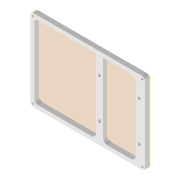
# Autodesk Inventor part: Omniscope_USBC_Base_Bottom
Saved by Autodesk Inventor 2022 (Build 260153000, 153)
## iProperties
Created: 2023-05-17
Part Number: Omniscope_USBC_Base_Bottom
Material: Generisch
Document SubType Name: Modeling
Designer: diederichbenedict
Density: 1 g/cm^3
Appearance: Vorgabe
Author: diederichbenedict
Autodesk Inventor part; units mm, degrees
(part 1 of 3)
ref_plane "YZ Plane" through (0, 0, 0) normal (1, 0, 0) x (0, 1, 0)
ref_plane "XZ Plane" through (0, 0, 0) normal (0, 1, 0) x (-1, 0, 0)
ref_plane "XY Plane" through (0, 0, 0) normal (0, 0, 1) x (1, 0, 0)
ref_plane "Arbeitsebene1" through (0, 0, 0) normal (0, 0, 1) x (1, 0, 0)
sketch "Skizze1" plane through (0, 0, 0) normal (0, 0, 1) x (1, 0, 0)
  line L0 (-66.421, 45.4152) -> (66.421, 45.4152)
  line L1 (-66.421, -45.4152) -> (-66.421, 45.4152)
  line L2 (66.421, -45.4152) -> (-66.421, -45.4152)
  line L3 (66.421, 45.4152) -> (66.421, -45.4152)
  line L4 (44.2834, -26.0546) -> (45.8834, -26.0546)
  line L5 (44.2834, -25.4046) -> (44.2834, -26.0546)
  line L6 (45.8834, -25.4046) -> (44.2834, -25.4046)
  line L7 (45.8834, -26.0546) -> (45.8834, -25.4046)
  line L8 (44.2834, -33.9546) -> (45.8834, -33.9546)
  line L9 (44.2834, -33.3046) -> (44.2834, -33.9546)
  line L10 (45.8834, -33.3046) -> (44.2834, -33.3046)
  line L11 (45.8834, -33.9546) -> (45.8834, -33.3046)
  line L12 (43.4184, -27.0796) -> (44.2084, -27.0796)
  line L13 (43.4184, -26.6796) -> (43.4184, -27.0796)
  line L14 (44.2084, -26.6796) -> (43.4184, -26.6796)
  line L15 (44.2084, -27.0796) -> (44.2084, -26.6796)
  line L16 (45.9584, -27.0796) -> (46.7484, -27.0796)
  line L17 (45.9584, -26.6796) -> (45.9584, -27.0796)
  line L18 (46.7484, -26.6796) -> (45.9584, -26.6796)
  line L19 (46.7484, -27.0796) -> (46.7484, -26.6796)
  line L20 (43.4184, -27.8796) -> (44.2084, -27.8796)
  line L21 (43.4184, -27.4796) -> (43.4184, -27.8796)
  line L22 (44.2084, -27.4796) -> (43.4184, -27.4796)
  line L23 (44.2084, -27.8796) -> (44.2084, -27.4796)
  line L24 (45.9584, -27.8796) -> (46.7484, -27.8796)
  line L25 (45.9584, -27.4796) -> (45.9584, -27.8796)
  line L26 (46.7484, -27.4796) -> (45.9584, -27.4796)
  line L27 (46.7484, -27.8796) -> (46.7484, -27.4796)
  line L28 (43.4184, -28.6796) -> (44.2084, -28.6796)
  line L29 (43.4184, -28.2796) -> (43.4184, -28.6796)
  line L30 (44.2084, -28.2796) -> (43.4184, -28.2796)
  line L31 (44.2084, -28.6796) -> (44.2084, -28.2796)
  line L32 (45.9584, -28.6796) -> (46.7484, -28.6796)
  line L33 (45.9584, -28.2796) -> (45.9584, -28.6796)
  line L34 (46.7484, -28.2796) -> (45.9584, -28.2796)
  line L35 (46.7484, -28.6796) -> (46.7484, -28.2796)
  line L36 (43.4184, -29.4796) -> (44.2084, -29.4796)
  line L37 (43.4184, -29.0796) -> (43.4184, -29.4796)
  line L38 (44.2084, -29.0796) -> (43.4184, -29.0796)
  line L39 (44.2084, -29.4796) -> (44.2084, -29.0796)
  line L40 (45.9584, -29.4796) -> (46.7484, -29.4796)
  line L41 (45.9584, -29.0796) -> (45.9584, -29.4796)
  line L42 (46.7484, -29.0796) -> (45.9584, -29.0796)
  line L43 (46.7484, -29.4796) -> (46.7484, -29.0796)
  line L44 (43.4184, -30.2796) -> (44.2084, -30.2796)
  line L45 (43.4184, -29.8796) -> (43.4184, -30.2796)
  line L46 (44.2084, -29.8796) -> (43.4184, -29.8796)
  line L47 (44.2084, -30.2796) -> (44.2084, -29.8796)
  line L48 (45.9584, -30.2796) -> (46.7484, -30.2796)
  line L49 (45.9584, -29.8796) -> (45.9584, -30.2796)
  line L50 (46.7484, -29.8796) -> (45.9584, -29.8796)
  line L51 (46.7484, -30.2796) -> (46.7484, -29.8796)
  line L52 (43.4184, -31.0796) -> (44.2084, -31.0796)
  line L53 (43.4184, -30.6796) -> (43.4184, -31.0796)
  line L54 (44.2084, -30.6796) -> (43.4184, -30.6796)
  line L55 (44.2084, -31.0796) -> (44.2084, -30.6796)
  line L56 (45.9584, -31.0796) -> (46.7484, -31.0796)
  line L57 (45.9584, -30.6796) -> (45.9584, -31.0796)
  line L58 (46.7484, -30.6796) -> (45.9584, -30.6796)
  line L59 (46.7484, -31.0796) -> (46.7484, -30.6796)
  line L60 (43.4184, -31.8796) -> (44.2084, -31.8796)
  line L61 (43.4184, -31.4796) -> (43.4184, -31.8796)
  line L62 (44.2084, -31.4796) -> (43.4184, -31.4796)
  line L63 (44.2084, -31.8796) -> (44.2084, -31.4796)
  line L64 (45.9584, -31.8796) -> (46.7484, -31.8796)
  line L65 (45.9584, -31.4796) -> (45.9584, -31.8796)
  line L66 (46.7484, -31.4796) -> (45.9584, -31.4796)
  line L67 (46.7484, -31.8796) -> (46.7484, -31.4796)
  line L68 (43.4184, -32.6796) -> (44.2084, -32.6796)
  line L69 (43.4184, -32.2796) -> (43.4184, -32.6796)
  line L70 (44.2084, -32.2796) -> (43.4184, -32.2796)
  line L71 (44.2084, -32.6796) -> (44.2084, -32.2796)
  line L72 (45.9584, -32.6796) -> (46.7484, -32.6796)
  line L73 (45.9584, -32.2796) -> (45.9584, -32.6796)
  line L74 (46.7484, -32.2796) -> (45.9584, -32.2796)
  line L75 (46.7484, -32.6796) -> (46.7484, -32.2796)
  line L76 (-29.4941, -14.7296) -> (-31.0941, -14.7296)
  line L77 (-29.4941, -15.3796) -> (-29.4941, -14.7296)
  line L78 (-31.0941, -15.3796) -> (-29.4941, -15.3796)
  line L79 (-31.0941, -14.7296) -> (-31.0941, -15.3796)
  line L80 (-29.4941, -6.8296) -> (-31.0941, -6.8296)
  line L81 (-29.4941, -7.4796) -> (-29.4941, -6.8296)
  line L82 (-31.0941, -7.4796) -> (-29.4941, -7.4796)
  line L83 (-31.0941, -6.8296) -> (-31.0941, -7.4796)
  line L84 (-28.6291, -13.7046) -> (-29.4191, -13.7046)
  line L85 (-28.6291, -14.1046) -> (-28.6291, -13.7046)
  line L86 (-29.4191, -14.1046) -> (-28.6291, -14.1046)
  line L87 (-29.4191, -13.7046) -> (-29.4191, -14.1046)
  line L88 (-31.1691, -13.7046) -> (-31.9591, -13.7046)
  line L89 (-31.1691, -14.1046) -> (-31.1691, -13.7046)
  line L90 (-31.9591, -14.1046) -> (-31.1691, -14.1046)
  line L91 (-31.9591, -13.7046) -> (-31.9591, -14.1046)
  line L92 (-28.6291, -12.9046) -> (-29.4191, -12.9046)
  line L93 (-28.6291, -13.3046) -> (-28.6291, -12.9046)
  line L94 (-29.4191, -13.3046) -> (-28.6291, -13.3046)
  line L95 (-29.4191, -12.9046) -> (-29.4191, -13.3046)
  line L96 (-31.1691, -12.9046) -> (-31.9591, -12.9046)
  line L97 (-31.1691, -13.3046) -> (-31.1691, -12.9046)
  line L98 (-31.9591, -13.3046) -> (-31.1691, -13.3046)
  line L99 (-31.9591, -12.9046) -> (-31.9591, -13.3046)
  line L100 (-28.6291, -12.1046) -> (-29.4191, -12.1046)
  line L101 (-28.6291, -12.5046) -> (-28.6291, -12.1046)
  line L102 (-29.4191, -12.5046) -> (-28.6291, -12.5046)
  line L103 (-29.4191, -12.1046) -> (-29.4191, -12.5046)
  line L104 (-31.1691, -12.1046) -> (-31.9591, -12.1046)
  line L105 (-31.1691, -12.5046) -> (-31.1691, -12.1046)
  line L106 (-31.9591, -12.5046) -> (-31.1691, -12.5046)
  line L107 (-31.9591, -12.1046) -> (-31.9591, -12.5046)
  line L108 (-28.6291, -11.3046) -> (-29.4191, -11.3046)
  line L109 (-28.6291, -11.7046) -> (-28.6291, -11.3046)
  line L110 (-29.4191, -11.7046) -> (-28.6291, -11.7046)
  line L111 (-29.4191, -11.3046) -> (-29.4191, -11.7046)
  line L112 (-31.1691, -11.3046) -> (-31.9591, -11.3046)
  line L113 (-31.1691, -11.7046) -> (-31.1691, -11.3046)
  line L114 (-31.9591, -11.7046) -> (-31.1691, -11.7046)
  line L115 (-31.9591, -11.3046) -> (-31.9591, -11.7046)
  line L116 (-28.6291, -10.5046) -> (-29.4191, -10.5046)
  line L117 (-28.6291, -10.9046) -> (-28.6291, -10.5046)
  line L118 (-29.4191, -10.9046) -> (-28.6291, -10.9046)
  line L119 (-29.4191, -10.5046) -> (-29.4191, -10.9046)
  line L120 (-31.1691, -10.5046) -> (-31.9591, -10.5046)
  line L121 (-31.1691, -10.9046) -> (-31.1691, -10.5046)
  line L122 (-31.9591, -10.9046) -> (-31.1691, -10.9046)
  line L123 (-31.9591, -10.5046) -> (-31.9591, -10.9046)
  line L124 (-28.6291, -9.7046) -> (-29.4191, -9.7046)
  line L125 (-28.6291, -10.1046) -> (-28.6291, -9.7046)
  line L126 (-29.4191, -10.1046) -> (-28.6291, -10.1046)
  line L127 (-29.4191, -9.7046) -> (-29.4191, -10.1046)
  line L128 (-31.1691, -9.7046) -> (-31.9591, -9.7046)
  line L129 (-31.1691, -10.1046) -> (-31.1691, -9.7046)
  line L130 (-31.9591, -10.1046) -> (-31.1691, -10.1046)
  line L131 (-31.9591, -9.7046) -> (-31.9591, -10.1046)
  line L132 (-28.6291, -8.9046) -> (-29.4191, -8.9046)
  line L133 (-28.6291, -9.3046) -> (-28.6291, -8.9046)
  line L134 (-29.4191, -9.3046) -> (-28.6291, -9.3046)
  line L135 (-29.4191, -8.9046) -> (-29.4191, -9.3046)
  line L136 (-31.1691, -8.9046) -> (-31.9591, -8.9046)
  line L137 (-31.1691, -9.3046) -> (-31.1691, -8.9046)
  line L138 (-31.9591, -9.3046) -> (-31.1691, -9.3046)
  line L139 (-31.9591, -8.9046) -> (-31.9591, -9.3046)
  line L140 (-28.6291, -8.1046) -> (-29.4191, -8.1046)
  line L141 (-28.6291, -8.5046) -> (-28.6291, -8.1046)
  line L142 (-29.4191, -8.5046) -> (-28.6291, -8.5046)
  line L143 (-29.4191, -8.1046) -> (-29.4191, -8.5046)
  line L144 (-31.1691, -8.1046) -> (-31.9591, -8.1046)
  line L145 (-31.1691, -8.5046) -> (-31.1691, -8.1046)
  line L146 (-31.9591, -8.5046) -> (-31.1691, -8.5046)
  line L147 (-31.9591, -8.1046) -> (-31.9591, -8.5046)
  line L148 (-10.6116, 22.9704) -> (-12.2116, 22.9704)
  line L149 (-10.6116, 22.3204) -> (-10.6116, 22.9704)
  line L150 (-12.2116, 22.3204) -> (-10.6116, 22.3204)
  line L151 (-12.2116, 22.9704) -> (-12.2116, 22.3204)
  line L152 (-10.6116, 30.8704) -> (-12.2116, 30.8704)
  line L153 (-10.6116, 30.2204) -> (-10.6116, 30.8704)
  line L154 (-12.2116, 30.2204) -> (-10.6116, 30.2204)
  line L155 (-12.2116, 30.8704) -> (-12.2116, 30.2204)
  line L156 (-9.7466, 23.9954) -> (-10.5366, 23.9954)
  line L157 (-9.7466, 23.5954) -> (-9.7466, 23.9954)
  line L158 (-10.5366, 23.5954) -> (-9.7466, 23.5954)
  line L159 (-10.5366, 23.9954) -> (-10.5366, 23.5954)
  line L160 (-12.2866, 23.9954) -> (-13.0766, 23.9954)
  line L161 (-12.2866, 23.5954) -> (-12.2866, 23.9954)
  line L162 (-13.0766, 23.5954) -> (-12.2866, 23.5954)
  line L163 (-13.0766, 23.9954) -> (-13.0766, 23.5954)
  line L164 (-9.7466, 24.7954) -> (-10.5366, 24.7954)
  line L165 (-9.7466, 24.3954) -> (-9.7466, 24.7954)
  line L166 (-10.5366, 24.3954) -> (-9.7466, 24.3954)
  line L167 (-10.5366, 24.7954) -> (-10.5366, 24.3954)
  line L168 (-12.2866, 24.7954) -> (-13.0766, 24.7954)
  line L169 (-12.2866, 24.3954) -> (-12.2866, 24.7954)
  line L170 (-13.0766, 24.3954) -> (-12.2866, 24.3954)
  line L171 (-13.0766, 24.7954) -> (-13.0766, 24.3954)
  line L172 (-9.7466, 25.5954) -> (-10.5366, 25.5954)
  line L173 (-9.7466, 25.1954) -> (-9.7466, 25.5954)
  line L174 (-10.5366, 25.1954) -> (-9.7466, 25.1954)
  line L175 (-10.5366, 25.5954) -> (-10.5366, 25.1954)
  line L176 (-12.2866, 25.5954) -> (-13.0766, 25.5954)
  line L177 (-12.2866, 25.1954) -> (-12.2866, 25.5954)
  line L178 (-13.0766, 25.1954) -> (-12.2866, 25.1954)
  line L179 (-13.0766, 25.5954) -> (-13.0766, 25.1954)
  line L180 (-9.7466, 26.3954) -> (-10.5366, 26.3954)
  line L181 (-9.7466, 25.9954) -> (-9.7466, 26.3954)
  line L182 (-10.5366, 25.9954) -> (-9.7466, 25.9954)
  line L183 (-10.5366, 26.3954) -> (-10.5366, 25.9954)
  line L184 (-12.2866, 26.3954) -> (-13.0766, 26.3954)
  line L185 (-12.2866, 25.9954) -> (-12.2866, 26.3954)
  line L186 (-13.0766, 25.9954) -> (-12.2866, 25.9954)
  line L187 (-13.0766, 26.3954) -> (-13.0766, 25.9954)
  line L188 (-9.7466, 27.1954) -> (-10.5366, 27.1954)
  line L189 (-9.7466, 26.7954) -> (-9.7466, 27.1954)
  line L190 (-10.5366, 26.7954) -> (-9.7466, 26.7954)
  line L191 (-10.5366, 27.1954) -> (-10.5366, 26.7954)
  line L192 (-12.2866, 27.1954) -> (-13.0766, 27.1954)
  line L193 (-12.2866, 26.7954) -> (-12.2866, 27.1954)
  line L194 (-13.0766, 26.7954) -> (-12.2866, 26.7954)
  line L195 (-13.0766, 27.1954) -> (-13.0766, 26.7954)
  line L196 (-9.7466, 27.9954) -> (-10.5366, 27.9954)
  line L197 (-9.7466, 27.5954) -> (-9.7466, 27.9954)
  line L198 (-10.5366, 27.5954) -> (-9.7466, 27.5954)
  line L199 (-10.5366, 27.9954) -> (-10.5366, 27.5954)
  line L200 (-12.2866, 27.9954) -> (-13.0766, 27.9954)
  line L201 (-12.2866, 27.5954) -> (-12.2866, 27.9954)
  line L202 (-13.0766, 27.5954) -> (-12.2866, 27.5954)
  line L203 (-13.0766, 27.9954) -> (-13.0766, 27.5954)
  line L204 (-9.7466, 28.7954) -> (-10.5366, 28.7954)
  line L205 (-9.7466, 28.3954) -> (-9.7466, 28.7954)
  line L206 (-10.5366, 28.3954) -> (-9.7466, 28.3954)
  line L207 (-10.5366, 28.7954) -> (-10.5366, 28.3954)
  line L208 (-12.2866, 28.7954) -> (-13.0766, 28.7954)
  line L209 (-12.2866, 28.3954) -> (-12.2866, 28.7954)
  line L210 (-13.0766, 28.3954) -> (-12.2866, 28.3954)
  line L211 (-13.0766, 28.7954) -> (-13.0766, 28.3954)
  line L212 (-9.7466, 29.5954) -> (-10.5366, 29.5954)
  line L213 (-9.7466, 29.1954) -> (-9.7466, 29.5954)
  line L214 (-10.5366, 29.1954) -> (-9.7466, 29.1954)
  line L215 (-10.5366, 29.5954) -> (-10.5366, 29.1954)
  line L216 (-12.2866, 29.5954) -> (-13.0766, 29.5954)
  line L217 (-12.2866, 29.1954) -> (-12.2866, 29.5954)
  line L218 (-13.0766, 29.1954) -> (-12.2866, 29.1954)
  line L219 (-13.0766, 29.5954) -> (-13.0766, 29.1954)
  line L220 (8.1884, -14.8046) -> (6.5884, -14.8046)
  line L221 (8.1884, -15.4546) -> (8.1884, -14.8046)
  line L222 (6.5884, -15.4546) -> (8.1884, -15.4546)
  line L223 (6.5884, -14.8046) -> (6.5884, -15.4546)
  line L224 (8.1884, -6.9046) -> (6.5884, -6.9046)
  line L225 (8.1884, -7.5546) -> (8.1884, -6.9046)
  line L226 (6.5884, -7.5546) -> (8.1884, -7.5546)
  line L227 (6.5884, -6.9046) -> (6.5884, -7.5546)
  line L228 (9.0534, -13.7796) -> (8.2634, -13.7796)
  line L229 (9.0534, -14.1796) -> (9.0534, -13.7796)
  line L230 (8.2634, -14.1796) -> (9.0534, -14.1796)
  line L231 (8.2634, -13.7796) -> (8.2634, -14.1796)
  line L232 (6.5134, -13.7796) -> (5.7234, -13.7796)
  line L233 (6.5134, -14.1796) -> (6.5134, -13.7796)
  line L234 (5.7234, -14.1796) -> (6.5134, -14.1796)
  line L235 (5.7234, -13.7796) -> (5.7234, -14.1796)
  line L236 (9.0534, -12.9796) -> (8.2634, -12.9796)
  line L237 (9.0534, -13.3796) -> (9.0534, -12.9796)
  line L238 (8.2634, -13.3796) -> (9.0534, -13.3796)
  line L239 (8.2634, -12.9796) -> (8.2634, -13.3796)
  line L240 (6.5134, -12.9796) -> (5.7234, -12.9796)
  line L241 (6.5134, -13.3796) -> (6.5134, -12.9796)
  line L242 (5.7234, -13.3796) -> (6.5134, -13.3796)
  line L243 (5.7234, -12.9796) -> (5.7234, -13.3796)
  line L244 (9.0534, -12.1796) -> (8.2634, -12.1796)
  line L245 (9.0534, -12.5796) -> (9.0534, -12.1796)
  line L246 (8.2634, -12.5796) -> (9.0534, -12.5796)
  line L247 (8.2634, -12.1796) -> (8.2634, -12.5796)
  line L248 (6.5134, -12.1796) -> (5.7234, -12.1796)
  line L249 (6.5134, -12.5796) -> (6.5134, -12.1796)
  line L250 (5.7234, -12.5796) -> (6.5134, -12.5796)
  line L251 (5.7234, -12.1796) -> (5.7234, -12.5796)
  line L252 (9.0534, -11.3796) -> (8.2634, -11.3796)
  line L253 (9.0534, -11.7796) -> (9.0534, -11.3796)
  line L254 (8.2634, -11.7796) -> (9.0534, -11.7796)
  line L255 (8.2634, -11.3796) -> (8.2634, -11.7796)
  line L256 (6.5134, -11.3796) -> (5.7234, -11.3796)
  line L257 (6.5134, -11.7796) -> (6.5134, -11.3796)
  line L258 (5.7234, -11.7796) -> (6.5134, -11.7796)
  line L259 (5.7234, -11.3796) -> (5.7234, -11.7796)
  line L260 (9.0534, -10.5796) -> (8.2634, -10.5796)
  line L261 (9.0534, -10.9796) -> (9.0534, -10.5796)
  line L262 (8.2634, -10.9796) -> (9.0534, -10.9796)
  line L263 (8.2634, -10.5796) -> (8.2634, -10.9796)
  line L264 (6.5134, -10.5796) -> (5.7234, -10.5796)
  line L265 (6.5134, -10.9796) -> (6.5134, -10.5796)
  line L266 (5.7234, -10.9796) -> (6.5134, -10.9796)
  line L267 (5.7234, -10.5796) -> (5.7234, -10.9796)
  line L268 (9.0534, -9.7796) -> (8.2634, -9.7796)
  line L269 (9.0534, -10.1796) -> (9.0534, -9.7796)
  line L270 (8.2634, -10.1796) -> (9.0534, -10.1796)
  line L271 (8.2634, -9.7796) -> (8.2634, -10.1796)
  line L272 (6.5134, -9.7796) -> (5.7234, -9.7796)
  line L273 (6.5134, -10.1796) -> (6.5134, -9.7796)
  line L274 (5.7234, -10.1796) -> (6.5134, -10.1796)
  line L275 (5.7234, -9.7796) -> (5.7234, -10.1796)
  line L276 (9.0534, -8.9796) -> (8.2634, -8.9796)
  line L277 (9.0534, -9.3796) -> (9.0534, -8.9796)
  line L278 (8.2634, -9.3796) -> (9.0534, -9.3796)
  line L279 (8.2634, -8.9796) -> (8.2634, -9.3796)
  line L280 (6.5134, -8.9796) -> (5.7234, -8.9796)
  line L281 (6.5134, -9.3796) -> (6.5134, -8.9796)
  line L282 (5.7234, -9.3796) -> (6.5134, -9.3796)
  line L283 (5.7234, -8.9796) -> (5.7234, -9.3796)
  line L284 (9.0534, -8.1796) -> (8.2634, -8.1796)
  line L285 (9.0534, -8.5796) -> (9.0534, -8.1796)
  line L286 (8.2634, -8.5796) -> (9.0534, -8.5796)
  line L287 (8.2634, -8.1796) -> (8.2634, -8.5796)
  line L288 (6.5134, -8.1796) -> (5.7234, -8.1796)
  line L289 (6.5134, -8.5796) -> (6.5134, -8.1796)
  line L290 (5.7234, -8.5796) -> (6.5134, -8.5796)
  line L291 (5.7234, -8.1796) -> (5.7234, -8.5796)
  line L292 (44.4409, 11.6204) -> (46.0409, 11.6204)
  line L293 (44.4409, 12.2704) -> (44.4409, 11.6204)
  line L294 (46.0409, 12.2704) -> (44.4409, 12.2704)
  line L295 (46.0409, 11.6204) -> (46.0409, 12.2704)
  line L296 (44.4409, 3.7204) -> (46.0409, 3.7204)
  line L297 (44.4409, 4.3704) -> (44.4409, 3.7204)
  line L298 (46.0409, 4.3704) -> (44.4409, 4.3704)
  line L299 (46.0409, 3.7204) -> (46.0409, 4.3704)
  line L300 (43.5759, 10.5954) -> (44.3659, 10.5954)
  line L301 (43.5759, 10.9954) -> (43.5759, 10.5954)
  line L302 (44.3659, 10.9954) -> (43.5759, 10.9954)
  line L303 (44.3659, 10.5954) -> (44.3659, 10.9954)
  line L304 (46.1159, 10.5954) -> (46.9059, 10.5954)
  line L305 (46.1159, 10.9954) -> (46.1159, 10.5954)
  line L306 (46.9059, 10.9954) -> (46.1159, 10.9954)
  line L307 (46.9059, 10.5954) -> (46.9059, 10.9954)
  line L308 (43.5759, 9.7954) -> (44.3659, 9.7954)
  line L309 (43.5759, 10.1954) -> (43.5759, 9.7954)
  line L310 (44.3659, 10.1954) -> (43.5759, 10.1954)
  line L311 (44.3659, 9.7954) -> (44.3659, 10.1954)
  line L312 (46.1159, 9.7954) -> (46.9059, 9.7954)
  line L313 (46.1159, 10.1954) -> (46.1159, 9.7954)
  line L314 (46.9059, 10.1954) -> (46.1159, 10.1954)
  line L315 (46.9059, 9.7954) -> (46.9059, 10.1954)
  line L316 (43.5759, 8.9954) -> (44.3659, 8.9954)
  line L317 (43.5759, 9.3954) -> (43.5759, 8.9954)
  line L318 (44.3659, 9.3954) -> (43.5759, 9.3954)
  line L319 (44.3659, 8.9954) -> (44.3659, 9.3954)
  line L320 (46.1159, 8.9954) -> (46.9059, 8.9954)
  line L321 (46.1159, 9.3954) -> (46.1159, 8.9954)
  line L322 (46.9059, 9.3954) -> (46.1159, 9.3954)
  line L323 (46.9059, 8.9954) -> (46.9059, 9.3954)
  line L324 (43.5759, 8.1954) -> (44.3659, 8.1954)
  line L325 (43.5759, 8.5954) -> (43.5759, 8.1954)
  line L326 (44.3659, 8.5954) -> (43.5759, 8.5954)
  line L327 (44.3659, 8.1954) -> (44.3659, 8.5954)
  line L328 (46.1159, 8.1954) -> (46.9059, 8.1954)
  line L329 (46.1159, 8.5954) -> (46.1159, 8.1954)
  line L330 (46.9059, 8.5954) -> (46.1159, 8.5954)
  line L331 (46.9059, 8.1954) -> (46.9059, 8.5954)
  line L332 (43.5759, 7.3954) -> (44.3659, 7.3954)
  line L333 (43.5759, 7.7954) -> (43.5759, 7.3954)
  line L334 (44.3659, 7.7954) -> (43.5759, 7.7954)
  line L335 (44.3659, 7.3954) -> (44.3659, 7.7954)
  line L336 (46.1159, 7.3954) -> (46.9059, 7.3954)
  line L337 (46.1159, 7.7954) -> (46.1159, 7.3954)
  line L338 (46.9059, 7.7954) -> (46.1159, 7.7954)
  line L339 (46.9059, 7.3954) -> (46.9059, 7.7954)
  line L340 (43.5759, 6.5954) -> (44.3659, 6.5954)
  line L341 (43.5759, 6.9954) -> (43.5759, 6.5954)
  line L342 (44.3659, 6.9954) -> (43.5759, 6.9954)
  line L343 (44.3659, 6.5954) -> (44.3659, 6.9954)
  line L344 (46.1159, 6.5954) -> (46.9059, 6.5954)
  line L345 (46.1159, 6.9954) -> (46.1159, 6.5954)
  line L346 (46.9059, 6.9954) -> (46.1159, 6.9954)
  line L347 (46.9059, 6.5954) -> (46.9059, 6.9954)
  line L348 (43.5759, 5.7954) -> (44.3659, 5.7954)
  line L349 (43.5759, 6.1954) -> (43.5759, 5.7954)
  line L350 (44.3659, 6.1954) -> (43.5759, 6.1954)
  line L351 (44.3659, 5.7954) -> (44.3659, 6.1954)
  line L352 (46.1159, 5.7954) -> (46.9059, 5.7954)
  line L353 (46.1159, 6.1954) -> (46.1159, 5.7954)
  line L354 (46.9059, 6.1954) -> (46.1159, 6.1954)
  line L355 (46.9059, 5.7954) -> (46.9059, 6.1954)
  line L356 (43.5759, 4.9954) -> (44.3659, 4.9954)
  line L357 (43.5759, 5.3954) -> (43.5759, 4.9954)
  line L358 (44.3659, 5.3954) -> (43.5759, 5.3954)
  line L359 (44.3659, 4.9954) -> (44.3659, 5.3954)
  line L360 (46.1159, 4.9954) -> (46.9059, 4.9954)
  line L361 (46.1159, 5.3954) -> (46.1159, 4.9954)
  line L362 (46.9059, 5.3954) -> (46.1159, 5.3954)
  line L363 (46.9059, 4.9954) -> (46.9059, 5.3954)
  line L364 (27.0884, 23.0704) -> (25.4884, 23.0704)
  line L365 (27.0884, 22.4204) -> (27.0884, 23.0704)
  line L366 (25.4884, 22.4204) -> (27.0884, 22.4204)
  line L367 (25.4884, 23.0704) -> (25.4884, 22.4204)
  line L368 (27.0884, 30.9704) -> (25.4884, 30.9704)
  line L369 (27.0884, 30.3204) -> (27.0884, 30.9704)
  line L370 (25.4884, 30.3204) -> (27.0884, 30.3204)
  line L371 (25.4884, 30.9704) -> (25.4884, 30.3204)
  line L372 (27.9534, 24.0954) -> (27.1634, 24.0954)
  line L373 (27.9534, 23.6954) -> (27.9534, 24.0954)
  line L374 (27.1634, 23.6954) -> (27.9534, 23.6954)
  line L375 (27.1634, 24.0954) -> (27.1634, 23.6954)
  line L376 (25.4134, 24.0954) -> (24.6234, 24.0954)
  line L377 (25.4134, 23.6954) -> (25.4134, 24.0954)
  line L378 (24.6234, 23.6954) -> (25.4134, 23.6954)
  line L379 (24.6234, 24.0954) -> (24.6234, 23.6954)
  line L380 (27.9534, 24.8954) -> (27.1634, 24.8954)
  line L381 (27.9534, 24.4954) -> (27.9534, 24.8954)
  line L382 (27.1634, 24.4954) -> (27.9534, 24.4954)
  line L383 (27.1634, 24.8954) -> (27.1634, 24.4954)
  line L384 (25.4134, 24.8954) -> (24.6234, 24.8954)
  line L385 (25.4134, 24.4954) -> (25.4134, 24.8954)
  line L386 (24.6234, 24.4954) -> (25.4134, 24.4954)
  line L387 (24.6234, 24.8954) -> (24.6234, 24.4954)
  line L388 (27.9534, 25.6954) -> (27.1634, 25.6954)
  line L389 (27.9534, 25.2954) -> (27.9534, 25.6954)
  line L390 (27.1634, 25.2954) -> (27.9534, 25.2954)
  line L391 (27.1634, 25.6954) -> (27.1634, 25.2954)
  line L392 (25.4134, 25.6954) -> (24.6234, 25.6954)
  line L393 (25.4134, 25.2954) -> (25.4134, 25.6954)
  line L394 (24.6234, 25.2954) -> (25.4134, 25.2954)
  line L395 (24.6234, 25.6954) -> (24.6234, 25.2954)
  line L396 (27.9534, 26.4954) -> (27.1634, 26.4954)
  line L397 (27.9534, 26.0954) -> (27.9534, 26.4954)
  line L398 (27.1634, 26.0954) -> (27.9534, 26.0954)
  line L399 (27.1634, 26.4954) -> (27.1634, 26.0954)
  line L400 (25.4134, 26.4954) -> (24.6234, 26.4954)
  line L401 (25.4134, 26.0954) -> (25.4134, 26.4954)
  line L402 (24.6234, 26.0954) -> (25.4134, 26.0954)
  line L403 (24.6234, 26.4954) -> (24.6234, 26.0954)
  line L404 (27.9534, 27.2954) -> (27.1634, 27.2954)
  line L405 (27.9534, 26.8954) -> (27.9534, 27.2954)
  line L406 (27.1634, 26.8954) -> (27.9534, 26.8954)
  line L407 (27.1634, 27.2954) -> (27.1634, 26.8954)
  line L408 (25.4134, 27.2954) -> (24.6234, 27.2954)
  line L409 (25.4134, 26.8954) -> (25.4134, 27.2954)
  line L410 (24.6234, 26.8954) -> (25.4134, 26.8954)
  line L411 (24.6234, 27.2954) -> (24.6234, 26.8954)
  line L412 (27.9534, 28.0954) -> (27.1634, 28.0954)
  line L413 (27.9534, 27.6954) -> (27.9534, 28.0954)
  line L414 (27.1634, 27.6954) -> (27.9534, 27.6954)
  line L415 (27.1634, 28.0954) -> (27.1634, 27.6954)
  line L416 (25.4134, 28.0954) -> (24.6234, 28.0954)
  line L417 (25.4134, 27.6954) -> (25.4134, 28.0954)
  line L418 (24.6234, 27.6954) -> (25.4134, 27.6954)
  line L419 (24.6234, 28.0954) -> (24.6234, 27.6954)
  line L420 (27.9534, 28.8954) -> (27.1634, 28.8954)
  line L421 (27.9534, 28.4954) -> (27.9534, 28.8954)
  line L422 (27.1634, 28.4954) -> (27.9534, 28.4954)
  line L423 (27.1634, 28.8954) -> (27.1634, 28.4954)
  line L424 (25.4134, 28.8954) -> (24.6234, 28.8954)
  line L425 (25.4134, 28.4954) -> (25.4134, 28.8954)
  line L426 (24.6234, 28.4954) -> (25.4134, 28.4954)
  line L427 (24.6234, 28.8954) -> (24.6234, 28.4954)
  line L428 (27.9534, 29.6954) -> (27.1634, 29.6954)
  line L429 (27.9534, 29.2954) -> (27.9534, 29.6954)
  line L430 (27.1634, 29.2954) -> (27.9534, 29.2954)
  line L431 (27.1634, 29.6954) -> (27.1634, 29.2954)
  line L432 (25.4134, 29.6954) -> (24.6234, 29.6954)
  line L433 (25.4134, 29.2954) -> (25.4134, 29.6954)
  line L434 (24.6234, 29.2954) -> (25.4134, 29.2954)
  line L435 (24.6234, 29.6954) -> (24.6234, 29.2954)
  line L436 (6.8784, 11.6704) -> (8.4784, 11.6704)
  line L437 (6.8784, 12.3204) -> (6.8784, 11.6704)
  line L438 (8.4784, 12.3204) -> (6.8784, 12.3204)
  line L439 (8.4784, 11.6704) -> (8.4784, 12.3204)
  line L440 (6.8784, 3.7704) -> (8.4784, 3.7704)
  line L441 (6.8784, 4.4204) -> (6.8784, 3.7704)
  line L442 (8.4784, 4.4204) -> (6.8784, 4.4204)
  line L443 (8.4784, 3.7704) -> (8.4784, 4.4204)
  line L444 (6.0134, 10.6454) -> (6.8034, 10.6454)
  line L445 (6.0134, 11.0454) -> (6.0134, 10.6454)
  line L446 (6.8034, 11.0454) -> (6.0134, 11.0454)
  line L447 (6.8034, 10.6454) -> (6.8034, 11.0454)
  line L448 (8.5534, 10.6454) -> (9.3434, 10.6454)
  line L449 (8.5534, 11.0454) -> (8.5534, 10.6454)
  line L450 (9.3434, 11.0454) -> (8.5534, 11.0454)
  line L451 (9.3434, 10.6454) -> (9.3434, 11.0454)
  line L452 (6.0134, 9.8454) -> (6.8034, 9.8454)
  line L453 (6.0134, 10.2454) -> (6.0134, 9.8454)
  line L454 (6.8034, 10.2454) -> (6.0134, 10.2454)
  line L455 (6.8034, 9.8454) -> (6.8034, 10.2454)
  line L456 (8.5534, 9.8454) -> (9.3434, 9.8454)
  line L457 (8.5534, 10.2454) -> (8.5534, 9.8454)
  line L458 (9.3434, 10.2454) -> (8.5534, 10.2454)
  line L459 (9.3434, 9.8454) -> (9.3434, 10.2454)
  line L460 (6.0134, 9.0454) -> (6.8034, 9.0454)
  line L461 (6.0134, 9.4454) -> (6.0134, 9.0454)
  line L462 (6.8034, 9.4454) -> (6.0134, 9.4454)
  line L463 (6.8034, 9.0454) -> (6.8034, 9.4454)
  line L464 (8.5534, 9.0454) -> (9.3434, 9.0454)
  line L465 (8.5534, 9.4454) -> (8.5534, 9.0454)
  line L466 (9.3434, 9.4454) -> (8.5534, 9.4454)
  line L467 (9.3434, 9.0454) -> (9.3434, 9.4454)
  line L468 (6.0134, 8.2454) -> (6.8034, 8.2454)
  line L469 (6.0134, 8.6454) -> (6.0134, 8.2454)
  line L470 (6.8034, 8.6454) -> (6.0134, 8.6454)
  line L471 (6.8034, 8.2454) -> (6.8034, 8.6454)
  line L472 (8.5534, 8.2454) -> (9.3434, 8.2454)
  line L473 (8.5534, 8.6454) -> (8.5534, 8.2454)
  line L474 (9.3434, 8.6454) -> (8.5534, 8.6454)
  line L475 (9.3434, 8.2454) -> (9.3434, 8.6454)
  line L476 (6.0134, 7.4454) -> (6.8034, 7.4454)
  line L477 (6.0134, 7.8454) -> (6.0134, 7.4454)
  line L478 (6.8034, 7.8454) -> (6.0134, 7.8454)
  line L479 (6.8034, 7.4454) -> (6.8034, 7.8454)
  line L480 (8.5534, 7.4454) -> (9.3434, 7.4454)
  line L481 (8.5534, 7.8454) -> (8.5534, 7.4454)
  line L482 (9.3434, 7.8454) -> (8.5534, 7.8454)
  line L483 (9.3434, 7.4454) -> (9.3434, 7.8454)
  line L484 (6.0134, 6.6454) -> (6.8034, 6.6454)
  line L485 (6.0134, 7.0454) -> (6.0134, 6.6454)
  line L486 (6.8034, 7.0454) -> (6.0134, 7.0454)
  line L487 (6.8034, 6.6454) -> (6.8034, 7.0454)
  line L488 (8.5534, 6.6454) -> (9.3434, 6.6454)
  line L489 (8.5534, 7.0454) -> (8.5534, 6.6454)
  line L490 (9.3434, 7.0454) -> (8.5534, 7.0454)
  line L491 (9.3434, 6.6454) -> (9.3434, 7.0454)
  line L492 (6.0134, 5.8454) -> (6.8034, 5.8454)
  line L493 (6.0134, 6.2454) -> (6.0134, 5.8454)
  line L494 (6.8034, 6.2454) -> (6.0134, 6.2454)
  line L495 (6.8034, 5.8454) -> (6.8034, 6.2454)
  line L496 (8.5534, 5.8454) -> (9.3434, 5.8454)
  line L497 (8.5534, 6.2454) -> (8.5534, 5.8454)
  line L498 (9.3434, 6.2454) -> (8.5534, 6.2454)
  line L499 (9.3434, 5.8454) -> (9.3434, 6.2454)
  line L500 (6.0134, 5.0454) -> (6.8034, 5.0454)
  line L501 (6.0134, 5.4454) -> (6.0134, 5.0454)
  line L502 (6.8034, 5.4454) -> (6.0134, 5.4454)
  line L503 (6.8034, 5.0454) -> (6.8034, 5.4454)
  line L504 (8.5534, 5.0454) -> (9.3434, 5.0454)
  line L505 (8.5534, 5.4454) -> (8.5534, 5.0454)
  line L506 (9.3434, 5.4454) -> (8.5534, 5.4454)
  line L507 (9.3434, 5.0454) -> (9.3434, 5.4454)
  line L508 (-49.8716, 11.5454) -> (-48.2716, 11.5454)
  line L509 (-49.8716, 12.1954) -> (-49.8716, 11.5454)
  line L510 (-48.2716, 12.1954) -> (-49.8716, 12.1954)
  line L511 (-48.2716, 11.5454) -> (-48.2716, 12.1954)
  line L512 (-49.8716, 3.6454) -> (-48.2716, 3.6454)
  line L513 (-49.8716, 4.2954) -> (-49.8716, 3.6454)
  line L514 (-48.2716, 4.2954) -> (-49.8716, 4.2954)
  line L515 (-48.2716, 3.6454) -> (-48.2716, 4.2954)
  line L516 (-50.7366, 10.5204) -> (-49.9466, 10.5204)
  line L517 (-50.7366, 10.9204) -> (-50.7366, 10.5204)
  line L518 (-49.9466, 10.9204) -> (-50.7366, 10.9204)
  line L519 (-49.9466, 10.5204) -> (-49.9466, 10.9204)
  line L520 (-48.1966, 10.5204) -> (-47.4066, 10.5204)
  line L521 (-48.1966, 10.9204) -> (-48.1966, 10.5204)
  line L522 (-47.4066, 10.9204) -> (-48.1966, 10.9204)
  line L523 (-47.4066, 10.5204) -> (-47.4066, 10.9204)
  line L524 (-50.7366, 9.7204) -> (-49.9466, 9.7204)
  line L525 (-50.7366, 10.1204) -> (-50.7366, 9.7204)
  line L526 (-49.9466, 10.1204) -> (-50.7366, 10.1204)
  line L527 (-49.9466, 9.7204) -> (-49.9466, 10.1204)
  line L528 (-48.1966, 9.7204) -> (-47.4066, 9.7204)
  line L529 (-48.1966, 10.1204) -> (-48.1966, 9.7204)
  line L530 (-47.4066, 10.1204) -> (-48.1966, 10.1204)
  line L531 (-47.4066, 9.7204) -> (-47.4066, 10.1204)
  line L532 (-50.7366, 8.9204) -> (-49.9466, 8.9204)
  line L533 (-50.7366, 9.3204) -> (-50.7366, 8.9204)
  line L534 (-49.9466, 9.3204) -> (-50.7366, 9.3204)
  line L535 (-49.9466, 8.9204) -> (-49.9466, 9.3204)
  line L536 (-48.1966, 8.9204) -> (-47.4066, 8.9204)
  line L537 (-48.1966, 9.3204) -> (-48.1966, 8.9204)
  line L538 (-47.4066, 9.3204) -> (-48.1966, 9.3204)
  line L539 (-47.4066, 8.9204) -> (-47.4066, 9.3204)
  line L540 (-50.7366, 8.1204) -> (-49.9466, 8.1204)
  line L541 (-50.7366, 8.5204) -> (-50.7366, 8.1204)
  line L542 (-49.9466, 8.5204) -> (-50.7366, 8.5204)
  line L543 (-49.9466, 8.1204) -> (-49.9466, 8.5204)
  line L544 (-48.1966, 8.1204) -> (-47.4066, 8.1204)
  line L545 (-48.1966, 8.5204) -> (-48.1966, 8.1204)
  line L546 (-47.4066, 8.5204) -> (-48.1966, 8.5204)
  line L547 (-47.4066, 8.1204) -> (-47.4066, 8.5204)
  line L548 (-50.7366, 7.3204) -> (-49.9466, 7.3204)
  line L549 (-50.7366, 7.7204) -> (-50.7366, 7.3204)
  line L550 (-49.9466, 7.7204) -> (-50.7366, 7.7204)
  line L551 (-49.9466, 7.3204) -> (-49.9466, 7.7204)
  line L552 (-48.1966, 7.3204) -> (-47.4066, 7.3204)
  line L553 (-48.1966, 7.7204) -> (-48.1966, 7.3204)
  line L554 (-47.4066, 7.7204) -> (-48.1966, 7.7204)
  line L555 (-47.4066, 7.3204) -> (-47.4066, 7.7204)
  line L556 (-50.7366, 6.5204) -> (-49.9466, 6.5204)
  line L557 (-50.7366, 6.9204) -> (-50.7366, 6.5204)
  line L558 (-49.9466, 6.9204) -> (-50.7366, 6.9204)
  line L559 (-49.9466, 6.5204) -> (-49.9466, 6.9204)
  line L560 (-48.1966, 6.5204) -> (-47.4066, 6.5204)
  line L561 (-48.1966, 6.9204) -> (-48.1966, 6.5204)
  line L562 (-47.4066, 6.9204) -> (-48.1966, 6.9204)
  line L563 (-47.4066, 6.5204) -> (-47.4066, 6.9204)
  line L564 (-50.7366, 5.7204) -> (-49.9466, 5.7204)
  line L565 (-50.7366, 6.1204) -> (-50.7366, 5.7204)
  line L566 (-49.9466, 6.1204) -> (-50.7366, 6.1204)
  line L567 (-49.9466, 5.7204) -> (-49.9466, 6.1204)
  line L568 (-48.1966, 5.7204) -> (-47.4066, 5.7204)
  line L569 (-48.1966, 6.1204) -> (-48.1966, 5.7204)
  line L570 (-47.4066, 6.1204) -> (-48.1966, 6.1204)
  line L571 (-47.4066, 5.7204) -> (-47.4066, 6.1204)
  line L572 (-50.7366, 4.9204) -> (-49.9466, 4.9204)
  line L573 (-50.7366, 5.3204) -> (-50.7366, 4.9204)
  line L574 (-49.9466, 5.3204) -> (-50.7366, 5.3204)
  line L575 (-49.9466, 4.9204) -> (-49.9466, 5.3204)
  line L576 (-48.1966, 4.9204) -> (-47.4066, 4.9204)
  line L577 (-48.1966, 5.3204) -> (-48.1966, 4.9204)
  line L578 (-47.4066, 5.3204) -> (-48.1966, 5.3204)
  line L579 (-47.4066, 4.9204) -> (-47.4066, 5.3204)
  line L580 (-29.4191, 23.0454) -> (-31.0191, 23.0454)
  line L581 (-29.4191, 22.3954) -> (-29.4191, 23.0454)
  line L582 (-31.0191, 22.3954) -> (-29.4191, 22.3954)
  line L583 (-31.0191, 23.0454) -> (-31.0191, 22.3954)
  line L584 (-29.4191, 30.9454) -> (-31.0191, 30.9454)
  line L585 (-29.4191, 30.2954) -> (-29.4191, 30.9454)
  line L586 (-31.0191, 30.2954) -> (-29.4191, 30.2954)
  line L587 (-31.0191, 30.9454) -> (-31.0191, 30.2954)
  line L588 (-28.5541, 24.0704) -> (-29.3441, 24.0704)
  line L589 (-28.5541, 23.6704) -> (-28.5541, 24.0704)
  line L590 (-29.3441, 23.6704) -> (-28.5541, 23.6704)
  line L591 (-29.3441, 24.0704) -> (-29.3441, 23.6704)
  line L592 (-31.0941, 24.0704) -> (-31.8841, 24.0704)
  line L593 (-31.0941, 23.6704) -> (-31.0941, 24.0704)
  line L594 (-31.8841, 23.6704) -> (-31.0941, 23.6704)
  line L595 (-31.8841, 24.0704) -> (-31.8841, 23.6704)
  line L596 (-28.5541, 24.8704) -> (-29.3441, 24.8704)
  line L597 (-28.5541, 24.4704) -> (-28.5541, 24.8704)
  line L598 (-29.3441, 24.4704) -> (-28.5541, 24.4704)
  line L599 (-29.3441, 24.8704) -> (-29.3441, 24.4704)
  line L600 (-31.0941, 24.8704) -> (-31.8841, 24.8704)
  line L601 (-31.0941, 24.4704) -> (-31.0941, 24.8704)
  line L602 (-31.8841, 24.4704) -> (-31.0941, 24.4704)
  line L603 (-31.8841, 24.8704) -> (-31.8841, 24.4704)
  line L604 (-28.5541, 25.6704) -> (-29.3441, 25.6704)
  line L605 (-28.5541, 25.2704) -> (-28.5541, 25.6704)
  line L606 (-29.3441, 25.2704) -> (-28.5541, 25.2704)
  line L607 (-29.3441, 25.6704) -> (-29.3441, 25.2704)
  line L608 (-31.0941, 25.6704) -> (-31.8841, 25.6704)
  line L609 (-31.0941, 25.2704) -> (-31.0941, 25.6704)
  line L610 (-31.8841, 25.2704) -> (-31.0941, 25.2704)
  line L611 (-31.8841, 25.6704) -> (-31.8841, 25.2704)
  line L612 (-28.5541, 26.4704) -> (-29.3441, 26.4704)
  line L613 (-28.5541, 26.0704) -> (-28.5541, 26.4704)
  line L614 (-29.3441, 26.0704) -> (-28.5541, 26.0704)
  line L615 (-29.3441, 26.4704) -> (-29.3441, 26.0704)
  line L616 (-31.0941, 26.4704) -> (-31.8841, 26.4704)
  line L617 (-31.0941, 26.0704) -> (-31.0941, 26.4704)
  line L618 (-31.8841, 26.0704) -> (-31.0941, 26.0704)
  line L619 (-31.8841, 26.4704) -> (-31.8841, 26.0704)
  line L620 (-28.5541, 27.2704) -> (-29.3441, 27.2704)
  line L621 (-28.5541, 26.8704) -> (-28.5541, 27.2704)
  line L622 (-29.3441, 26.8704) -> (-28.5541, 26.8704)
  line L623 (-29.3441, 27.2704) -> (-29.3441, 26.8704)
  line L624 (-31.0941, 27.2704) -> (-31.8841, 27.2704)
  line L625 (-31.0941, 26.8704) -> (-31.0941, 27.2704)
  line L626 (-31.8841, 26.8704) -> (-31.0941, 26.8704)
  line L627 (-31.8841, 27.2704) -> (-31.8841, 26.8704)
  line L628 (-28.5541, 28.0704) -> (-29.3441, 28.0704)
  line L629 (-28.5541, 27.6704) -> (-28.5541, 28.0704)
  line L630 (-29.3441, 27.6704) -> (-28.5541, 27.6704)
  line L631 (-29.3441, 28.0704) -> (-29.3441, 27.6704)
  line L632 (-31.0941, 28.0704) -> (-31.8841, 28.0704)
  line L633 (-31.0941, 27.6704) -> (-31.0941, 28.0704)
  line L634 (-31.8841, 27.6704) -> (-31.0941, 27.6704)
  line L635 (-31.8841, 28.0704) -> (-31.8841, 27.6704)
  line L636 (-28.5541, 28.8704) -> (-29.3441, 28.8704)
  line L637 (-28.5541, 28.4704) -> (-28.5541, 28.8704)
  line L638 (-29.3441, 28.4704) -> (-28.5541, 28.4704)
  line L639 (-29.3441, 28.8704) -> (-29.3441, 28.4704)
  line L640 (-31.0941, 28.8704) -> (-31.8841, 28.8704)
  line L641 (-31.0941, 28.4704) -> (-31.0941, 28.8704)
  line L642 (-31.8841, 28.4704) -> (-31.0941, 28.4704)
  line L643 (-31.8841, 28.8704) -> (-31.8841, 28.4704)
  line L644 (-28.5541, 29.6704) -> (-29.3441, 29.6704)
  line L645 (-28.5541, 29.2704) -> (-28.5541, 29.6704)
  line L646 (-29.3441, 29.2704) -> (-28.5541, 29.2704)
  line L647 (-29.3441, 29.6704) -> (-29.3441, 29.2704)
  line L648 (-31.0941, 29.6704) -> (-31.8841, 29.6704)
  line L649 (-31.0941, 29.2704) -> (-31.0941, 29.6704)
  line L650 (-31.8841, 29.2704) -> (-31.0941, 29.2704)
  line L651 (-31.8841, 29.6704) -> (-31.8841, 29.2704)
  line L652 (-48.1741, 23.0204) -> (-49.7741, 23.0204)
  line L653 (-48.1741, 22.3704) -> (-48.1741, 23.0204)
  line L654 (-49.7741, 22.3704) -> (-48.1741, 22.3704)
  line L655 (-49.7741, 23.0204) -> (-49.7741, 22.3704)
  line L656 (-48.1741, 30.9204) -> (-49.7741, 30.9204)
  line L657 (-48.1741, 30.2704) -> (-48.1741, 30.9204)
  line L658 (-49.7741, 30.2704) -> (-48.1741, 30.2704)
  line L659 (-49.7741, 30.9204) -> (-49.7741, 30.2704)
  line L660 (-47.3091, 24.0454) -> (-48.0991, 24.0454)
  line L661 (-47.3091, 23.6454) -> (-47.3091, 24.0454)
  line L662 (-48.0991, 23.6454) -> (-47.3091, 23.6454)
  line L663 (-48.0991, 24.0454) -> (-48.0991, 23.6454)
  line L664 (-49.8491, 24.0454) -> (-50.6391, 24.0454)
  line L665 (-49.8491, 23.6454) -> (-49.8491, 24.0454)
  line L666 (-50.6391, 23.6454) -> (-49.8491, 23.6454)
  line L667 (-50.6391, 24.0454) -> (-50.6391, 23.6454)
  line L668 (-47.3091, 24.8454) -> (-48.0991, 24.8454)
  line L669 (-47.3091, 24.4454) -> (-47.3091, 24.8454)
  line L670 (-48.0991, 24.4454) -> (-47.3091, 24.4454)
  line L671 (-48.0991, 24.8454) -> (-48.0991, 24.4454)
  line L672 (-49.8491, 24.8454) -> (-50.6391, 24.8454)
  line L673 (-49.8491, 24.4454) -> (-49.8491, 24.8454)
  line L674 (-50.6391, 24.4454) -> (-49.8491, 24.4454)
  line L675 (-50.6391, 24.8454) -> (-50.6391, 24.4454)
  line L676 (-47.3091, 25.6454) -> (-48.0991, 25.6454)
  line L677 (-47.3091, 25.2454) -> (-47.3091, 25.6454)
  line L678 (-48.0991, 25.2454) -> (-47.3091, 25.2454)
  line L679 (-48.0991, 25.6454) -> (-48.0991, 25.2454)
  line L680 (-49.8491, 25.6454) -> (-50.6391, 25.6454)
  line L681 (-49.8491, 25.2454) -> (-49.8491, 25.6454)
  line L682 (-50.6391, 25.2454) -> (-49.8491, 25.2454)
  line L683 (-50.6391, 25.6454) -> (-50.6391, 25.2454)
  line L684 (-47.3091, 26.4454) -> (-48.0991, 26.4454)
  line L685 (-47.3091, 26.0454) -> (-47.3091, 26.4454)
  line L686 (-48.0991, 26.0454) -> (-47.3091, 26.0454)
  line L687 (-48.0991, 26.4454) -> (-48.0991, 26.0454)
  line L688 (-49.8491, 26.4454) -> (-50.6391, 26.4454)
  line L689 (-49.8491, 26.0454) -> (-49.8491, 26.4454)
  line L690 (-50.6391, 26.0454) -> (-49.8491, 26.0454)
  line L691 (-50.6391, 26.4454) -> (-50.6391, 26.0454)
  line L692 (-47.3091, 27.2454) -> (-48.0991, 27.2454)
  line L693 (-47.3091, 26.8454) -> (-47.3091, 27.2454)
  line L694 (-48.0991, 26.8454) -> (-47.3091, 26.8454)
  line L695 (-48.0991, 27.2454) -> (-48.0991, 26.8454)
  line L696 (-49.8491, 27.2454) -> (-50.6391, 27.2454)
  line L697 (-49.8491, 26.8454) -> (-49.8491, 27.2454)
  line L698 (-50.6391, 26.8454) -> (-49.8491, 26.8454)
  line L699 (-50.6391, 27.2454) -> (-50.6391, 26.8454)
  line L700 (-47.3091, 28.0454) -> (-48.0991, 28.0454)
  line L701 (-47.3091, 27.6454) -> (-47.3091, 28.0454)
  line L702 (-48.0991, 27.6454) -> (-47.3091, 27.6454)
  line L703 (-48.0991, 28.0454) -> (-48.0991, 27.6454)
  line L704 (-49.8491, 28.0454) -> (-50.6391, 28.0454)
  line L705 (-49.8491, 27.6454) -> (-49.8491, 28.0454)
  line L706 (-50.6391, 27.6454) -> (-49.8491, 27.6454)
  line L707 (-50.6391, 28.0454) -> (-50.6391, 27.6454)
  line L708 (-47.3091, 28.8454) -> (-48.0991, 28.8454)
  line L709 (-47.3091, 28.4454) -> (-47.3091, 28.8454)
  line L710 (-48.0991, 28.4454) -> (-47.3091, 28.4454)
  line L711 (-48.0991, 28.8454) -> (-48.0991, 28.4454)
  line L712 (-49.8491, 28.8454) -> (-50.6391, 28.8454)
  line L713 (-49.8491, 28.4454) -> (-49.8491, 28.8454)
  line L714 (-50.6391, 28.4454) -> (-49.8491, 28.4454)
  line L715 (-50.6391, 28.8454) -> (-50.6391, 28.4454)
  line L716 (-47.3091, 29.6454) -> (-48.0991, 29.6454)
  line L717 (-47.3091, 29.2454) -> (-47.3091, 29.6454)
  line L718 (-48.0991, 29.2454) -> (-47.3091, 29.2454)
  line L719 (-48.0991, 29.6454) -> (-48.0991, 29.2454)
  line L720 (-49.8491, 29.6454) -> (-50.6391, 29.6454)
  line L721 (-49.8491, 29.2454) -> (-49.8491, 29.6454)
  line L722 (-50.6391, 29.2454) -> (-49.8491, 29.2454)
  line L723 (-50.6391, 29.6454) -> (-50.6391, 29.2454)
  line L724 (27.0134, -14.7046) -> (25.4134, -14.7046)
  line L725 (27.0134, -15.3546) -> (27.0134, -14.7046)
  line L726 (25.4134, -15.3546) -> (27.0134, -15.3546)
  line L727 (25.4134, -14.7046) -> (25.4134, -15.3546)
  line L728 (27.0134, -6.8046) -> (25.4134, -6.8046)
  line L729 (27.0134, -7.4546) -> (27.0134, -6.8046)
  line L730 (25.4134, -7.4546) -> (27.0134, -7.4546)
  line L731 (25.4134, -6.8046) -> (25.4134, -7.4546)
  line L732 (27.8784, -13.6796) -> (27.0884, -13.6796)
  line L733 (27.8784, -14.0796) -> (27.8784, -13.6796)
  line L734 (27.0884, -14.0796) -> (27.8784, -14.0796)
  line L735 (27.0884, -13.6796) -> (27.0884, -14.0796)
  line L736 (25.3384, -13.6796) -> (24.5484, -13.6796)
  line L737 (25.3384, -14.0796) -> (25.3384, -13.6796)
  line L738 (24.5484, -14.0796) -> (25.3384, -14.0796)
  line L739 (24.5484, -13.6796) -> (24.5484, -14.0796)
  line L740 (27.8784, -12.8796) -> (27.0884, -12.8796)
  line L741 (27.8784, -13.2796) -> (27.8784, -12.8796)
  line L742 (27.0884, -13.2796) -> (27.8784, -13.2796)
  line L743 (27.0884, -12.8796) -> (27.0884, -13.2796)
  line L744 (25.3384, -12.8796) -> (24.5484, -12.8796)
  line L745 (25.3384, -13.2796) -> (25.3384, -12.8796)
  line L746 (24.5484, -13.2796) -> (25.3384, -13.2796)
  line L747 (24.5484, -12.8796) -> (24.5484, -13.2796)
  line L748 (27.8784, -12.0796) -> (27.0884, -12.0796)
  line L749 (27.8784, -12.4796) -> (27.8784, -12.0796)
  line L750 (27.0884, -12.4796) -> (27.8784, -12.4796)
  line L751 (27.0884, -12.0796) -> (27.0884, -12.4796)
  line L752 (25.3384, -12.0796) -> (24.5484, -12.0796)
  line L753 (25.3384, -12.4796) -> (25.3384, -12.0796)
  line L754 (24.5484, -12.4796) -> (25.3384, -12.4796)
  line L755 (24.5484, -12.0796) -> (24.5484, -12.4796)
  line L756 (27.8784, -11.2796) -> (27.0884, -11.2796)
  line L757 (27.8784, -11.6796) -> (27.8784, -11.2796)
  line L758 (27.0884, -11.6796) -> (27.8784, -11.6796)
  line L759 (27.0884, -11.2796) -> (27.0884, -11.6796)
  line L760 (25.3384, -11.2796) -> (24.5484, -11.2796)
  line L761 (25.3384, -11.6796) -> (25.3384, -11.2796)
  line L762 (24.5484, -11.6796) -> (25.3384, -11.6796)
  line L763 (24.5484, -11.2796) -> (24.5484, -11.6796)
  line L764 (27.8784, -10.4796) -> (27.0884, -10.4796)
  line L765 (27.8784, -10.8796) -> (27.8784, -10.4796)
  line L766 (27.0884, -10.8796) -> (27.8784, -10.8796)
  line L767 (27.0884, -10.4796) -> (27.0884, -10.8796)
  line L768 (25.3384, -10.4796) -> (24.5484, -10.4796)
  line L769 (25.3384, -10.8796) -> (25.3384, -10.4796)
  line L770 (24.5484, -10.8796) -> (25.3384, -10.8796)
  line L771 (24.5484, -10.4796) -> (24.5484, -10.8796)
  line L772 (27.8784, -9.6796) -> (27.0884, -9.6796)
  line L773 (27.8784, -10.0796) -> (27.8784, -9.6796)
  line L774 (27.0884, -10.0796) -> (27.8784, -10.0796)
  line L775 (27.0884, -9.6796) -> (27.0884, -10.0796)
  line L776 (25.3384, -9.6796) -> (24.5484, -9.6796)
  line L777 (25.3384, -10.0796) -> (25.3384, -9.6796)
  line L778 (24.5484, -10.0796) -> (25.3384, -10.0796)
  line L779 (24.5484, -9.6796) -> (24.5484, -10.0796)
  line L780 (27.8784, -8.8796) -> (27.0884, -8.8796)
  line L781 (27.8784, -9.2796) -> (27.8784, -8.8796)
  line L782 (27.0884, -9.2796) -> (27.8784, -9.2796)
  line L783 (27.0884, -8.8796) -> (27.0884, -9.2796)
  line L784 (25.3384, -8.8796) -> (24.5484, -8.8796)
  line L785 (25.3384, -9.2796) -> (25.3384, -8.8796)
  line L786 (24.5484, -9.2796) -> (25.3384, -9.2796)
  line L787 (24.5484, -8.8796) -> (24.5484, -9.2796)
  line L788 (27.8784, -8.0796) -> (27.0884, -8.0796)
  line L789 (27.8784, -8.4796) -> (27.8784, -8.0796)
  line L790 (27.0884, -8.4796) -> (27.8784, -8.4796)
  line L791 (27.0884, -8.0796) -> (27.0884, -8.4796)
  line L792 (25.3384, -8.0796) -> (24.5484, -8.0796)
  line L793 (25.3384, -8.4796) -> (25.3384, -8.0796)
  line L794 (24.5484, -8.4796) -> (25.3384, -8.4796)
  line L795 (24.5484, -8.0796) -> (24.5484, -8.4796)
  line L796 (-12.1541, -26.0046) -> (-10.5541, -26.0046)
  line L797 (-12.1541, -25.3546) -> (-12.1541, -26.0046)
  line L798 (-10.5541, -25.3546) -> (-12.1541, -25.3546)
  line L799 (-10.5541, -26.0046) -> (-10.5541, -25.3546)
  line L800 (-12.1541, -33.9046) -> (-10.5541, -33.9046)
  line L801 (-12.1541, -33.2546) -> (-12.1541, -33.9046)
  line L802 (-10.5541, -33.2546) -> (-12.1541, -33.2546)
  line L803 (-10.5541, -33.9046) -> (-10.5541, -33.2546)
  line L804 (-13.0191, -27.0296) -> (-12.2291, -27.0296)
  line L805 (-13.0191, -26.6296) -> (-13.0191, -27.0296)
  line L806 (-12.2291, -26.6296) -> (-13.0191, -26.6296)
  line L807 (-12.2291, -27.0296) -> (-12.2291, -26.6296)
  line L808 (-10.4791, -27.0296) -> (-9.6891, -27.0296)
  line L809 (-10.4791, -26.6296) -> (-10.4791, -27.0296)
  line L810 (-9.6891, -26.6296) -> (-10.4791, -26.6296)
  line L811 (-9.6891, -27.0296) -> (-9.6891, -26.6296)
  line L812 (-13.0191, -27.8296) -> (-12.2291, -27.8296)
  line L813 (-13.0191, -27.4296) -> (-13.0191, -27.8296)
  line L814 (-12.2291, -27.4296) -> (-13.0191, -27.4296)
  line L815 (-12.2291, -27.8296) -> (-12.2291, -27.4296)
  line L816 (-10.4791, -27.8296) -> (-9.6891, -27.8296)
  line L817 (-10.4791, -27.4296) -> (-10.4791, -27.8296)
  line L818 (-9.6891, -27.4296) -> (-10.4791, -27.4296)
  line L819 (-9.6891, -27.8296) -> (-9.6891, -27.4296)
  line L820 (-13.0191, -28.6296) -> (-12.2291, -28.6296)
  line L821 (-13.0191, -28.2296) -> (-13.0191, -28.6296)
  line L822 (-12.2291, -28.2296) -> (-13.0191, -28.2296)
  line L823 (-12.2291, -28.6296) -> (-12.2291, -28.2296)
  line L824 (-10.4791, -28.6296) -> (-9.6891, -28.6296)
  line L825 (-10.4791, -28.2296) -> (-10.4791, -28.6296)
  line L826 (-9.6891, -28.2296) -> (-10.4791, -28.2296)
  line L827 (-9.6891, -28.6296) -> (-9.6891, -28.2296)
  line L828 (-13.0191, -29.4296) -> (-12.2291, -29.4296)
  line L829 (-13.0191, -29.0296) -> (-13.0191, -29.4296)
  line L830 (-12.2291, -29.0296) -> (-13.0191, -29.0296)
  line L831 (-12.2291, -29.4296) -> (-12.2291, -29.0296)
  line L832 (-10.4791, -29.4296) -> (-9.6891, -29.4296)
  line L833 (-10.4791, -29.0296) -> (-10.4791, -29.4296)
  line L834 (-9.6891, -29.0296) -> (-10.4791, -29.0296)
  line L835 (-9.6891, -29.4296) -> (-9.6891, -29.0296)
  line L836 (-13.0191, -30.2296) -> (-12.2291, -30.2296)
  line L837 (-13.0191, -29.8296) -> (-13.0191, -30.2296)
  line L838 (-12.2291, -29.8296) -> (-13.0191, -29.8296)
  line L839 (-12.2291, -30.2296) -> (-12.2291, -29.8296)
  line L840 (-10.4791, -30.2296) -> (-9.6891, -30.2296)
  line L841 (-10.4791, -29.8296) -> (-10.4791, -30.2296)
  line L842 (-9.6891, -29.8296) -> (-10.4791, -29.8296)
  line L843 (-9.6891, -30.2296) -> (-9.6891, -29.8296)
  line L844 (-13.0191, -31.0296) -> (-12.2291, -31.0296)
  line L845 (-13.0191, -30.6296) -> (-13.0191, -31.0296)
  line L846 (-12.2291, -30.6296) -> (-13.0191, -30.6296)
  line L847 (-12.2291, -31.0296) -> (-12.2291, -30.6296)
  line L848 (-10.4791, -31.0296) -> (-9.6891, -31.0296)
  line L849 (-10.4791, -30.6296) -> (-10.4791, -31.0296)
  line L850 (-9.6891, -30.6296) -> (-10.4791, -30.6296)
  line L851 (-9.6891, -31.0296) -> (-9.6891, -30.6296)
  line L852 (-13.0191, -31.8296) -> (-12.2291, -31.8296)
  line L853 (-13.0191, -31.4296) -> (-13.0191, -31.8296)
  line L854 (-12.2291, -31.4296) -> (-13.0191, -31.4296)
  line L855 (-12.2291, -31.8296) -> (-12.2291, -31.4296)
  line L856 (-10.4791, -31.8296) -> (-9.6891, -31.8296)
  line L857 (-10.4791, -31.4296) -> (-10.4791, -31.8296)
  line L858 (-9.6891, -31.4296) -> (-10.4791, -31.4296)
  line L859 (-9.6891, -31.8296) -> (-9.6891, -31.4296)
  line L860 (-13.0191, -32.6296) -> (-12.2291, -32.6296)
  line L861 (-13.0191, -32.2296) -> (-13.0191, -32.6296)
  line L862 (-12.2291, -32.2296) -> (-13.0191, -32.2296)
  line L863 (-12.2291, -32.6296) -> (-12.2291, -32.2296)
  line L864 (-10.4791, -32.6296) -> (-9.6891, -32.6296)
  line L865 (-10.4791, -32.2296) -> (-10.4791, -32.6296)
  line L866 (-9.6891, -32.2296) -> (-10.4791, -32.2296)
  line L867 (-9.6891, -32.6296) -> (-9.6891, -32.2296)
  line L868 (-30.8216, 11.5704) -> (-29.2216, 11.5704)
  line L869 (-30.8216, 12.2204) -> (-30.8216, 11.5704)
  line L870 (-29.2216, 12.2204) -> (-30.8216, 12.2204)
  line L871 (-29.2216, 11.5704) -> (-29.2216, 12.2204)
  line L872 (-30.8216, 3.6704) -> (-29.2216, 3.6704)
  line L873 (-30.8216, 4.3204) -> (-30.8216, 3.6704)
  line L874 (-29.2216, 4.3204) -> (-30.8216, 4.3204)
  line L875 (-29.2216, 3.6704) -> (-29.2216, 4.3204)
  line L876 (-31.6866, 10.5454) -> (-30.8966, 10.5454)
  line L877 (-31.6866, 10.9454) -> (-31.6866, 10.5454)
  line L878 (-30.8966, 10.9454) -> (-31.6866, 10.9454)
  line L879 (-30.8966, 10.5454) -> (-30.8966, 10.9454)
  line L880 (-29.1466, 10.5454) -> (-28.3566, 10.5454)
  line L881 (-29.1466, 10.9454) -> (-29.1466, 10.5454)
  line L882 (-28.3566, 10.9454) -> (-29.1466, 10.9454)
  line L883 (-28.3566, 10.5454) -> (-28.3566, 10.9454)
  line L884 (-31.6866, 9.7454) -> (-30.8966, 9.7454)
  line L885 (-31.6866, 10.1454) -> (-31.6866, 9.7454)
  line L886 (-30.8966, 10.1454) -> (-31.6866, 10.1454)
  line L887 (-30.8966, 9.7454) -> (-30.8966, 10.1454)
  line L888 (-29.1466, 9.7454) -> (-28.3566, 9.7454)
  line L889 (-29.1466, 10.1454) -> (-29.1466, 9.7454)
  line L890 (-28.3566, 10.1454) -> (-29.1466, 10.1454)
  line L891 (-28.3566, 9.7454) -> (-28.3566, 10.1454)
  line L892 (-31.6866, 8.9454) -> (-30.8966, 8.9454)
  line L893 (-31.6866, 9.3454) -> (-31.6866, 8.9454)
  line L894 (-30.8966, 9.3454) -> (-31.6866, 9.3454)
  line L895 (-30.8966, 8.9454) -> (-30.8966, 9.3454)
  line L896 (-29.1466, 8.9454) -> (-28.3566, 8.9454)
  line L897 (-29.1466, 9.3454) -> (-29.1466, 8.9454)
  line L898 (-28.3566, 9.3454) -> (-29.1466, 9.3454)
  line L899 (-28.3566, 8.9454) -> (-28.3566, 9.3454)
  line L900 (-31.6866, 8.1454) -> (-30.8966, 8.1454)
  line L901 (-31.6866, 8.5454) -> (-31.6866, 8.1454)
  line L902 (-30.8966, 8.5454) -> (-31.6866, 8.5454)
  line L903 (-30.8966, 8.1454) -> (-30.8966, 8.5454)
  line L904 (-29.1466, 8.1454) -> (-28.3566, 8.1454)
  line L905 (-29.1466, 8.5454) -> (-29.1466, 8.1454)
  line L906 (-28.3566, 8.5454) -> (-29.1466, 8.5454)
  line L907 (-28.3566, 8.1454) -> (-28.3566, 8.5454)
  line L908 (-31.6866, 7.3454) -> (-30.8966, 7.3454)
  line L909 (-31.6866, 7.7454) -> (-31.6866, 7.3454)
  line L910 (-30.8966, 7.7454) -> (-31.6866, 7.7454)
  line L911 (-30.8966, 7.3454) -> (-30.8966, 7.7454)
  line L912 (-29.1466, 7.3454) -> (-28.3566, 7.3454)
  line L913 (-29.1466, 7.7454) -> (-29.1466, 7.3454)
  line L914 (-28.3566, 7.7454) -> (-29.1466, 7.7454)
  line L915 (-28.3566, 7.3454) -> (-28.3566, 7.7454)